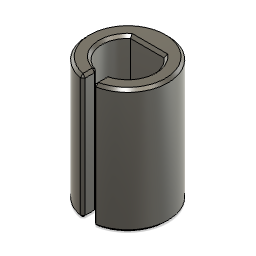
Motor Coupler v2 (Autodesk Fusion 360 design; units mm, degrees)
Autodesk Fusion 360 part; units mm, degrees
sketch "Sketch1" plane through (0, 0, 0) normal (0, 1, 0) x (1, 0, 0) in component "Coupler"
  circle A0 centre (0, 0) radius 3.9
  circle A1 centre (0, 0) radius 2.5
  line L0 (0, 0) -> (0, 1.9) construction
  line L1 (0, 1.9) -> (1.624808, 1.9)
  line L2 (0, 1.9) -> (-1.624808, 1.9)
  line L3 (0, 0) -> (0, -1.666667) construction
  line L4 (0, -1.666667) -> (0.5, -1.666667) construction
  line L5 (0, -1.666667) -> (-0.5, -1.666667) construction
  line L6 (0.5, -1.666667) -> (0.5, -3.867816)
  line L7 (-0.5, -1.666667) -> (-0.5, -3.867816)
  dimension "d6" = 7.8
  dimension "d7" = 5
  dimension "d8" = 1.9
  dimension "d9" = 1.666667
  dimension "d10" = 0.5
  dimension "d11" = 0.5
  constraint coincident A0.centre A1.centre
  constraint concentric A0 A1
  constraint vertical L0
  constraint perpendicular L0 L1
  constraint perpendicular L0 L2
  constraint parallel L0 L3
  constraint perpendicular L3 L4
  constraint perpendicular L3 L5
  constraint perpendicular L4 L6
  constraint perpendicular L5 L7
  measures "d6" diameter of A0
  measures "d7" diameter of A1
  measures "d8" distance of A0.centre L0.end
extrude "Extrude1" add sketch "Sketch1" along normal blind 12 contours A0 A1 L6 L7 | A1 L1 L2 picked at (-1.17588, -3.21813) picked at (0.117521, 2.291672) in component "Coupler"
chamfer "Chamfer1" distance 0.25 angle 45 4 faces at (0.850625, 12, -2.529404) (0.850625, 0, -2.529404) (-0.5, 4, 2.922265) (0.5, 4, 2.922265) in component "Coupler"
component "Coupler" placed x (1, 0, 0) y (0, 1, 0) z (0, 0, 1) at (0, 0, 0)
equation "MotorShaftDiameter = 5 mm"
equation "MotorShaftKeyDiameter = 4.4 mm"
equation "CouplerDiameter = 7.8 mm"
equation "CouplerHeight = 12 mm"
equation "Gap = 1 mm"
equation "d6 = CouplerDiameter"
equation "d7 = MotorShaftDiameter"
equation "d8 = MotorShaftKeyDiameter - MotorShaftDiameter / 2"
equation "d9 = MotorShaftDiameter / 3"
equation "d10 = Gap / 2"
equation "d11 = d10"
equation "d12 = CouplerHeight"
named bodies: "GR Motor Coupler"
